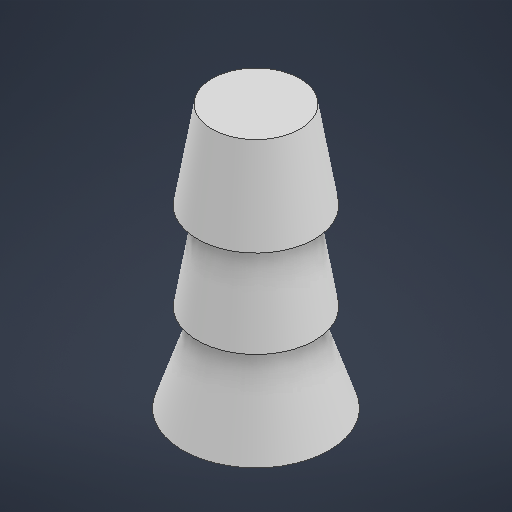
# Autodesk Inventor part: Valve_Plug_V1
Saved by Autodesk Inventor 2026.2 (Build 302298000, 298)
## iProperties
Created: 2026-01-25
Part Number: Valve_Plug_V1
Material: Generic
Document SubType Name: Modeling
Designer: vckot
Density: 1 g/cm^3
Appearance: Default
Author: vckot
Autodesk Inventor part; units mm, degrees
ref_plane "YZ Plane" through (0, 0, 0) normal (1, 0, 0) x (0, 1, 0)
ref_plane "XZ Plane" through (0, 0, 0) normal (0, 1, 0) x (-1, 0, 0)
ref_plane "XY Plane" through (0, 0, 0) normal (0, 0, 1) x (1, 0, 0)
sketch "Sketch1" plane through (0, 0, 0) normal (0, 0, 1) x (1, 0, 0)
  line L0 (-1.5, 0) -> (1.5, 0)
  line L1 (-2, -3) -> (2, -3)
  line L2 (-1.5, -3) -> (1.5, -3)
  line L3 (-2, -6) -> (2, -6)
  line L4 (-2, -6) -> (2, -6) construction
  line L5 (-1.5, -6) -> (1.5, -6)
  line L6 (-2.5, -9) -> (2.5, -9)
  line L7 (-1.5, 0) -> (-2, -3)
  line L8 (1.5, 0) -> (2, -3)
  line L9 (-1.5, -3) -> (-1.5, -3)
  line L10 (1.5, -3) -> (1.5, -3)
  line L11 (-2, -6) -> (-1.5, -3)
  line L12 (1.5, -3) -> (2, -6)
  line L13 (-1.5, -6) -> (-1.5, -6)
  line L14 (1.5, -6) -> (1.5, -6)
  line L15 (-1.5, -6) -> (-2.5, -9)
  line L16 (1.5, -6) -> (2.5, -9)
  line L17 (0, 0) -> (0, -9)
  point P0 (0, -6)
  point P1 (0, -6)
  dimension "d0" = 3
  dimension "d1" = 4
  dimension "d2" = 3
  dimension "d3" = 4
  dimension "d5" = 5
  dimension "d6" = 3
  dimension "d7" = 3
  dimension "d8" = 3
  dimension "d9" = 0
  dimension "d10" = 3
  dimension "d11" = 0
  dimension "d12" = 9
  constraints: 36 end point, 7 horizontal, 6 point on line, 4 midpoint, 3 vertical alignment, 2 equal length, 2 perpendicular, 1 parallel, 1 vertical
  measures "d0" distance of L0.start L0.end
  measures "d1" distance of L1.start L1.end
  measures "d2" distance of L2.start L2.end
  measures "d3" distance of L3.start L3.end
  measures "d5" distance of L6.start L6.end
  measures "d6" distance of L5.start L5.end
  measures "d7" distance between parallel lines of L0 L1
  measures "d8" distance between parallel lines of L5 L6
  measures "d9" distance between parallel lines of L3 L5
  measures "d10" distance between parallel lines of L3 L2
  measures "d11" distance between parallel lines of L1 L2
  measures "d12" distance between parallel lines of L6 L0
revolve "Revolution1" add sketch "Sketch1" angle 360 about axis through (0, 0, 0) along (0, -1, 0) contours L0 L8 L1 L17 | L1 L12 L3 L17 | L3 L16 L6 L17
body "Solid1"
